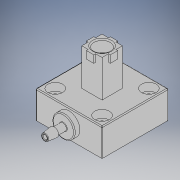
# Autodesk Inventor part: 9mm_ball_holder
Saved by Autodesk Inventor 2019 (Build 230136000, 136)
## iProperties
Created: 2019-03-11
Part Number: 9mm_ball_holder
Material: Generic
Document SubType Name: Modeling
Designer: Wilson Lab
Density: 1 g/cm^3
Appearance: Default
Author: Wilson Lab
Autodesk Inventor part; units mm, degrees
ref_plane "YZ Plane" through (0, 0, 0) normal (1, 0, 0) x (0, 1, 0)
ref_plane "XZ Plane" through (0, 0, 0) normal (0, 1, 0) x (-1, 0, 0)
ref_plane "XY Plane" through (0, 0, 0) normal (0, 0, 1) x (1, 0, 0)
sketch "Sketch1" plane through (0, 0, 0) normal (0, 0, 1) x (1, 0, 0)
  line L0 (0, 0) -> (-5.5, 0) construction
  line L1 (-5.5, 0) -> (-5.5, 20) construction
  line L2 (-5.5, 20) -> (0, 20) construction
  line L3 (0, 20) -> (0, 0) construction
  circle A0 centre (0, 20.35) radius 4.5 construction
  line L4 (-5.5, 20) -> (-5.1335, 20)
  line L5 (-0.75, 15.3188) -> (-0.75, 0)
  arc A1 (-4.4001, 19.4071) -> (-1.2857, 16.0376) centre (0, 20.35) ccw
  arc A2 (-0.75, 15.3188) -> (-1.2857, 16.0376) centre (-1.5, 15.3188) ccw
  arc A3 (-4.4001, 19.4071) -> (-5.1335, 20) centre (-5.1335, 19.25) ccw
  line L6 (-5.5, 20) -> (-5.5, 0)
  line L7 (-5.5, 0) -> (-0.75, 0)
  point P0 (-4.4864, 20)
  point P1 (-0.75, 15.9129)
  dimension "d1" = 20
  dimension "d5" = 9
  dimension "d6" = 0.35
  dimension "d7" = 0.75
  dimension "d8" = 0.75
  dimension "d9" = 0.75
  dimension "d133" = 5.5
  dimension "d134" = 1.0136
  constraints: 18 end point, 10 point on circle, 5 point on line, 4 centre point, 4 tangent, 3 perpendicular, 2 parallel, 1 collinear, 1 concentric, 1 horizontal
  measures "d1" distance between parallel lines of L0 L2
  measures "d5" diameter of A0
  measures "d6" distance of A0.centre L2.end
  measures "d7" distance between parallel lines of L3 L5
  measures "d8" radius of A2
  measures "d9" radius of A3
  measures "d133" distance between parallel lines of L1 L3
  measures "d134" distance of A0.start L1.end
revolve "Revolution1" add sketch "Sketch1" angle 360 about axis through (0, 20, 0) along (0, -1, 0)
ref_plane "Work Plane1" through (0, 20, 0) normal (0, 1, 0) x (1, 0, 0)
sketch "Sketch2" plane through (0, 20, 0) normal (0, 1, 0) x (1, 0, 0)
  circle A0 centre (0, 0) radius 5.5 projected
  circle A1 centre (0, 0) radius 5.5 construction
  line L0 (-5.5, -5.5) -> (5.5, -5.5)
  line L1 (5.5, -5.5) -> (5.5, 5.5)
  line L2 (5.5, 5.5) -> (-5.5, 5.5)
  line L3 (-5.5, 5.5) -> (-5.5, -5.5)
  circle A2 centre (0, 0) radius 1.2857 projected
  line L4 (-5.5, -5.5) -> (5.5, 5.5) construction
  line L5 (5.5, -5.5) -> (-5.5, 5.5) construction
  point P0 (0, 0)
  dimension "d124" = 0
  constraints: 12 end point, 2 midpoint, 2 parallel, 2 tangent, 1 centre point, 1 coincident, 1 horizontal, 1 perpendicular
  measures "d124" distance edge to line of A0 L1
extrude "Extrusion1" add sketch "Sketch2" against normal up to surface (20 mm away) contours L1 L0 A0 | A0 L2 L1 | A0 L3 L2 | L0 L3 A0
ref_plane "Work Plane7" through (0, 0, 0) normal (0, -1, 0) x (1, 0, 0)
sketch "Sketch11" plane through (0, 0, 0) normal (0, -1, 0) x (1, 0, 0)
  line L0 (0, 18) -> (0, 0) construction
  line L1 (-18, -18) -> (18, -18)
  line L2 (18, -18) -> (18, 18)
  line L3 (18, 18) -> (-18, 18)
  line L4 (-18, 18) -> (-18, -18)
  line L5 (-18, -18) -> (18, 18) construction
  line L6 (18, -18) -> (-18, 18) construction
  dimension "d60" = 36
  dimension "d61" = 36
  constraints: 14 end point, 3 midpoint, 2 parallel, 1 horizontal, 1 perpendicular
  measures "d60" distance of L1.end L2.end
  measures "d61" distance of L2.end L3.end
extrude "Extrusion6" add sketch "Sketch11" along normal blind 15
sketch "Sketch16" plane through (-18, 0, -18) normal (-1, 0, 0) x (0, 0, 1)
  line L0 (36, 0) -> (0, 0) construction
  line L1 (0, 0) -> (0, -15) construction
  line L2 (36, -15) -> (0, -15) construction
  line L3 (36, 0) -> (36, -15) construction
  line L4 (18.75, 15.3188) -> (18.75, 0) construction
  line L5 (17.25, 15.3188) -> (17.25, 0) construction
  line L6 (18, -7.5) -> (18, 0) construction
  line L7 (36, 0) -> (36, -15) construction
  line L8 (36, 0) -> (36, -7.5) construction
  line L9 (18, -7.5) -> (36, -7.5) construction
  circle A0 centre (18, -7.5) radius 4.225
  dimension "d64" = 8.45
  constraints: 6 end point, 1 centre point, 1 coincident, 1 horizontal, 1 midpoint, 1 vertical
  measures "d64" diameter of A0
extrude "Extrusion7" cut sketch "Sketch16" against normal blind 32.7
sketch "Sketch17" plane through (0, 0, 0) normal (0, -1, 0) x (1, 0, 0)
  circle A0 centre (0, 0) radius 0.75 projected
  point P0 (0, 0)
ref_plane "Work Plane8" through (-18, 0, 0) normal (0, 0, 1) x (1, 0, 0)
sketch "Sketch18" plane through (-18, 0, 0) normal (0, 0, 1) x (1, 0, 0)
  line L0 (18, 0) -> (18, -10.576)
  line L1 (0, -11.725) -> (32.7, -11.725) projected
  constraints: 2 end point, 1 vertical
sweep "Sweep3" cut profiles "Sketch17" path "Sketch18" path curves L0
fillet "Fillet1" radius 3 1 edges at (-0.75, -3.275, -0.001)
sketch "Sketch19" plane through (0, 0, 0) normal (0, 1, 0) x (1, 0, 0)
  line L0 (18, -18) -> (-18, -18) construction
  line L1 (18, 18) -> (18, -18) construction
  line L2 (-18, 18) -> (18, 18) construction
  line L3 (-18, -18) -> (-18, 18) construction
  line L4 (-12.7, 12.7) -> (12.7, 12.7) construction
  line L5 (12.7, 12.7) -> (12.7, -12.7) construction
  line L6 (12.7, -12.7) -> (-12.7, -12.7) construction
  line L7 (-12.7, -12.7) -> (-12.7, 12.7) construction
  circle A0 centre (0, 0) radius 1.2857 construction
  line L8 (-12.7, 12.7) -> (12.7, -12.7) construction
  line L9 (12.7, 12.7) -> (-12.7, -12.7) construction
  point P0 (0, 0)
  dimension "d70" = 25.4
  dimension "d71" = 25.4
  constraints: 12 end point, 4 coincident, 2 midpoint, 2 parallel, 1 horizontal, 1 perpendicular
  measures "d70" distance of L4.end L5.end
  measures "d71" distance of L5.end L6.end
hole "Hole3" at (12.7, 0, -12.7) at (12.7, 0, 12.7) at (-12.7, 0, 12.7) at (-12.7, 0, -12.7) direction (0, -1, 0) diameter 4.496 end through all counterbore diameter 7.938 counterbore depth 4.166
sketch "Sketch21" plane through (-18, 0, 0) normal (0, 0, 1) x (1, 0, 0)
  line L0 (0, -11.725) -> (0, -3.275) construction
  line L1 (0, 0) -> (0, -15) construction
  line L2 (0, -7.5) -> (-3, -7.5)
  line L3 (-3, -9.6296) -> (-3, -13.5)
  line L4 (-3, -13.5) -> (0, -13.5)
  line L5 (0, -13.5) -> (0, -7.5) construction
  line L6 (-3.25, -9.3796) -> (-8, -9.3796)
  arc A0 (-3, -9.6296) -> (-3.25, -9.3796) centre (-3.25, -9.6296) ccw
  line L7 (-8, -9.3796) -> (-8, -9.913)
  line L8 (-8, -9.913) -> (-12.8561, -9.4031)
  line L9 (-8, -9.3796) -> (-13.08, -9.3796) construction
  line L10 (-12.83, -8.65) -> (0, -8.65)
  line L11 (-13.08, -8.9) -> (-13.08, -9.1545)
  arc A1 (-12.83, -8.65) -> (-13.08, -8.9) centre (-12.83, -8.9) ccw
  arc A2 (-13.08, -9.1545) -> (-12.8561, -9.4031) centre (-12.83, -9.1545) ccw
  line L12 (0, -8.65) -> (0, -13.5)
  point P0 (18, 0)
  point P1 (-3, -9.3796)
  dimension "d79" = 3
  dimension "d80" = 6
  dimension "d81" = 5
  dimension "d82" = 1.8796
  dimension "d83" = 0.25
  dimension "d84" = 2.413
  dimension "d85" = 5.08
  dimension "d86" = 1.15
  dimension "d87" = 0.25
  dimension "d88" = 0.25
  constraints: 22 end point, 6 point on circle, 6 point on line, 6 tangent, 3 centre point, 3 horizontal, 2 parallel, 2 perpendicular, 2 vertical, 1 collinear, 1 midpoint
  measures "d79" distance of L3.end L4.end
  measures "d80" distance between parallel lines of L2 L4
  measures "d81" distance of point (-3, -9.38) L6.end
  measures "d82" distance between parallel lines of L2 L6
  measures "d83" radius of A0
  measures "d84" distance from line of L2 L7.end
  measures "d85" horizontal distance of L7.end L9.end
  measures "d86" distance between parallel lines of L10 L2
  measures "d87" radius of A1
  measures "d88" radius of A2
revolve "Revolution2" add sketch "Sketch21" angle 360 about axis through (-18, -7.5, 0) along (-1, 0, 0)
fillet "Fillet2" radius 0.5 9 edges at (-21, -1.5, 0) (0, 0, -18) (-18, 0, 0) (0, 0, 18) (18, 0, 0) (18, -7.5, 18) (-18, -7.5, 18) (-18, -7.5, -18) (18, -7.5, -18)
sketch "Sketch28" plane through (-5.5, 20, -5.5) normal (-1, 0, 0) x (0, 0, 1)
  line L0 (0, -20) -> (11, -20) construction
  line L1 (11, 0) -> (11, -20) construction
  line L2 (0, 0) -> (11, 0) construction
  line L3 (0, 0) -> (0, -20) construction
  line L4 (3.5, -4) -> (7.5, -4)
  line L5 (7.5, -4) -> (7.5, 0)
  line L6 (7.5, 0) -> (3.5, 0)
  line L7 (3.5, 0) -> (3.5, -4)
  line L8 (3.5, -2) -> (0, -2) construction
  line L9 (7.5, -2) -> (11, -2) construction
  point P0 (5.5, -20)
  dimension "d125" = 0
  dimension "d126" = 4
  constraints: 12 end point, 3 point on line, 2 equal length, 2 midpoint, 2 parallel, 2 perpendicular, 1 horizontal
  measures "d125" distance between parallel lines of L2 L6
  measures "d126" distance of L4.end L5.end
extrude "Extrusion13" add sketch "Sketch28" along normal blind 1
pattern_circular "Circular Pattern1" count 4 over 360 about axis through (0, -10, 0) along (0, 1, 0) of "Extrusion13"
body "Solid1"
